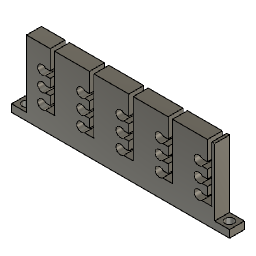
ESC Tray Holder v2 (Autodesk Fusion 360 design; units mm, degrees)
Autodesk Fusion 360 part; units mm, degrees
box "BoxPrimitive2" add length 25.4 width 76.2 height 2.54 placed x (0, 0, 1) y (1, 0, 0) z (0, 1, 0) at (0, 0, 0)
sketch "Sketch3" plane through (0, 2.54, 0) normal (0, 1, 0) x (-1, 0, 0)
  line L0 (0, 25.4) -> (-76.2, 25.4)
  line L1 (-76.2, 25.4) -> (-76.2, 0)
  line L2 (-76.2, 0) -> (0, 0)
  line L3 (0, 0) -> (0, 25.4)
  line L4 (-76.2, 12.7) -> (-72.39, 12.7)
  line L5 (-72.39, 12.7) -> (-72.39, 25.4)
  line L6 (-72.39, 25.4) -> (-69.215, 25.4)
  line L7 (-69.215, 25.4) -> (-69.215, 0)
  line L8 (-69.215, 0) -> (-72.39, 0)
  line L9 (-72.39, 12.7) -> (-72.39, 0)
  line L10 (-69.215, 12.7) -> (-59.055, 12.7)
  line L11 (-59.055, 12.7) -> (-59.055, 25.4)
  line L12 (-59.055, 25.4) -> (-55.88, 25.4)
  line L13 (-55.88, 25.4) -> (-55.88, 0)
  line L14 (-55.88, 0) -> (-59.055, 0)
  line L15 (-59.055, 12.7) -> (-59.055, 0)
  line L16 (-55.88, 12.7) -> (-45.72, 12.7)
  line L17 (-45.72, 12.7) -> (-45.72, 0)
  line L18 (-45.72, 0) -> (-42.545, 0)
  line L19 (-42.545, 0) -> (-42.545, 25.4)
  line L20 (-42.545, 25.4) -> (-45.72, 25.4)
  line L21 (-45.72, 12.7) -> (-45.72, 25.4)
  line L22 (-42.545, 12.7) -> (-32.385, 12.7)
  line L23 (-32.385, 12.7) -> (-32.385, 25.4)
  line L24 (-32.385, 25.4) -> (-29.21, 25.4)
  line L25 (-29.21, 25.4) -> (-29.21, 0)
  line L26 (-29.21, 0) -> (-32.385, 0)
  line L27 (-32.385, 0) -> (-32.385, 12.7)
  line L28 (-29.21, 12.7) -> (-19.05, 12.7)
  line L29 (-19.05, 12.7) -> (-19.05, 25.4)
  line L30 (-19.05, 25.4) -> (-15.875, 25.4)
  line L31 (-15.875, 25.4) -> (-15.875, 0)
  line L32 (-15.875, 0) -> (-19.05, 0)
  line L33 (-19.05, 0) -> (-19.05, 12.7)
  line L34 (-15.875, 12.7) -> (-12.065, 12.7)
  line L35 (-12.065, 12.7) -> (-12.065, 25.4)
  line L36 (-12.065, 12.7) -> (-12.065, 0)
  line L37 (-76.2, 12.7) -> (-76.2, 17.78)
  circle A0 centre (-70.8025, 17.78) radius 1.5875
  line L38 (-76.2, 12.7) -> (-76.2, 7.62)
  circle A1 centre (-70.8025, 7.62) radius 1.5875
  circle A2 centre (-70.8025, 12.7) radius 1.5875
  line L39 (-57.4675, 25.4) -> (-57.4675, 0)
  circle A3 centre (-57.4675, 12.7) radius 1.5875
  circle A4 centre (-57.4675, 17.78) radius 1.5875
  circle A5 centre (-57.4675, 7.62) radius 1.5875
  line L40 (-44.1325, 25.4) -> (-44.1325, 0)
  circle A6 centre (-44.1325, 12.7) radius 1.5875
  circle A7 centre (-44.1325, 17.78) radius 1.5875
  circle A8 centre (-44.1325, 7.62) radius 1.5875
  line L41 (-30.7975, 25.4) -> (-30.7975, 0)
  circle A9 centre (-30.7975, 12.7) radius 1.5875
  circle A10 centre (-30.7975, 7.62) radius 1.5875
  circle A11 centre (-30.7975, 17.78) radius 1.5875
  line L42 (-17.4625, 25.4) -> (-17.4625, 0)
  circle A12 centre (-17.4625, 12.7) radius 1.5875
  circle A13 centre (-17.4625, 17.78) radius 1.5875
  circle A14 centre (-17.4625, 7.62) radius 1.5875
  dimension "d17" = 3.81
  dimension "d18" = 3.175
  dimension "d19" = 3.175
  dimension "d20" = 10.16
  dimension "d21" = 3.175
  dimension "d22" = 3.175
  dimension "d23" = 10.16
  dimension "d24" = 3.175
  dimension "d25" = 3.175
  dimension "d26" = 10.16
  dimension "d27" = 3.175
  dimension "d28" = 3.175
  dimension "d29" = 10.16
  dimension "d30" = 3.175
  dimension "d31" = 3.175
  dimension "d32" = 3.81
  dimension "d37" = 5.08
  dimension "d38" = 3.175
  dimension "d39" = 5.08
  dimension "d40" = 3.175
  dimension "d41" = 3.175
  dimension "d42" = 3.175
  dimension "d43" = 3.175
  dimension "d44" = 3.175
  dimension "d45" = 3.175
  dimension "d46" = 3.175
  dimension "d47" = 3.175
  dimension "d48" = 3.175
  dimension "d49" = 3.175
  dimension "d50" = 3.175
  dimension "d51" = 3.175
  dimension "d52" = 3.175
  dimension "d53" = 3.175
  constraint midpoint L1 L4.start
  constraint perpendicular L1 L4
  constraint coincident L0 L5.end
  constraint perpendicular L0 L5
  constraint perpendicular L5 L6
  constraint coincident L2 L7.end
  constraint perpendicular L2 L7
  constraint perpendicular L7 L8
  constraint midpoint L7 L10.start
  constraint perpendicular L7 L10
  constraint coincident L0 L11.end
  constraint perpendicular L0 L11
  constraint coincident L0 L12.end
  constraint coincident L2 L13.end
  constraint perpendicular L2 L13
  constraint perpendicular L13 L14
  constraint midpoint L13 L16.start
  constraint perpendicular L13 L16
  constraint coincident L2 L17.end
  constraint perpendicular L14 L17
  constraint coincident L2 L18.end
  constraint coincident L0 L19.end
  constraint perpendicular L0 L19
  constraint perpendicular L19 L20
  constraint midpoint L19 L22.start
  constraint perpendicular L19 L22
  constraint coincident L0 L23.end
  constraint perpendicular L0 L23
  constraint coincident L0 L24.end
  constraint coincident L2 L25.end
  constraint perpendicular L2 L25
  constraint perpendicular L25 L26
  constraint midpoint L25 L28.start
  constraint perpendicular L25 L28
  constraint perpendicular L28 L29
  constraint perpendicular L29 L30
  constraint coincident L2 L31.end
  constraint perpendicular L2 L31
  constraint perpendicular L31 L32
  constraint midpoint L31 L34.start
  constraint perpendicular L31 L34
  constraint coincident L0 L35.end
  constraint perpendicular L0 L35
  constraint coincident L2 L36.end
  constraint perpendicular L2 L36
  constraint perpendicular L4 L37
  constraint perpendicular L4 L38
  constraint midpoint L12 L39.start
  constraint midpoint L14 L39.end
  constraint midpoint L39 A3.centre
  constraint coincident L39 A4.centre
  constraint coincident L39 A5.centre
  constraint midpoint L20 L40.start
  constraint midpoint L18 L40.end
  constraint midpoint L40 A6.centre
  constraint coincident L40 A7.centre
  constraint coincident L40 A8.centre
  constraint midpoint L24 L41.start
  constraint midpoint L26 L41.end
  constraint midpoint L41 A9.centre
  constraint coincident L41 A10.centre
  constraint coincident L41 A11.centre
  constraint midpoint L30 L42.start
  constraint midpoint L32 L42.end
  constraint midpoint L42 A12.centre
  constraint coincident L42 A13.centre
  constraint coincident L42 A14.centre
  measures "d17" distance of L4.start L4.end
  measures "d18" distance of L5.end L6.end
  measures "d19" distance of L7.end L8.end
  measures "d20" distance of L10.start L10.end
  measures "d21" distance of L11.end L12.end
  measures "d22" distance of L13.end L14.end
  measures "d23" distance of L16.start L16.end
  measures "d24" distance of L17.end L18.end
  measures "d25" distance of L19.end L20.end
  measures "d26" distance of L22.start L22.end
  measures "d27" distance of L23.end L24.end
  measures "d28" distance of L25.end L26.end
  measures "d29" distance of L28.start L28.end
  measures "d30" distance of L29.end L30.end
  measures "d31" distance of L31.end L32.end
  measures "d32" distance of L34.start L34.end
  measures "d37" distance of L4.start L37.end
  measures "d38" diameter of A0
  measures "d39" distance of L4.start L38.end
  measures "d40" diameter of A1
  measures "d41" diameter of A2
  measures "d42" diameter of A3
  measures "d43" diameter of A4
  measures "d44" diameter of A5
  measures "d45" diameter of A6
  measures "d46" diameter of A7
  measures "d47" diameter of A8
  measures "d48" diameter of A9
  measures "d49" diameter of A10
  measures "d50" diameter of A11
  measures "d51" diameter of A12
  measures "d52" diameter of A13
  measures "d53" diameter of A14
scale "Scale1" factors (0.841667, 1, 1) about (0, 2.54, 25.4) bodies 1
move_body "Move1" bodies 1 to x (1, 0, 0) y (0, 1, 0) z (0, 0, 1) at (12.065, 0, 0)
extrude "Extrude1" cut sketch "Sketch3" against normal blind 12.7 contours L42 A13 | L42 A12 | L42 A13 | L42 A14 | L42 A12 | L42 A14 | L41 A11 | L41 A9 | L41 A11 | L41 A10 | L41 A9 | L41 A10 | L40 A7 | L40 A6 | L40 A7 | L40 A8 | L40 A6 | L40 A8 | L39 A4 | L39 A3 | L39 A4 | L39 A5 | L39 A3 | L39 A5 | A0 | A2 | A1
sketch "Sketch4" plane through (76.2, 0, 0) normal (1, 0, 0) x (0, 1, 0)
  line L0 (2.54, 25.4) -> (0, 25.4)
  line L1 (0, 25.4) -> (0, 0)
  line L2 (0, 0) -> (2.54, 0)
  line L3 (2.54, 0) -> (2.54, 25.4)
  line L4 (2.54, 0) -> (2.54, 2.54)
  line L5 (0, 2.54) -> (2.54, 2.54)
  line L6 (0, 2.54) -> (0, 0)
  line L7 (2.54, 0) -> (0, 0)
  dimension "d56" = 2.54
  constraint coincident L2.end L3.start
  constraint coincident L3 L4.end
  constraint coincident L1 L5.start
  constraint perpendicular L4 L5
  constraint coincident L1.end L2.start
  measures "d56" distance of L2.end L4.end
extrude "Extrude2" add sketch "Sketch4" along normal blind 5.08 contours L1 L2 L3 L4 L5 L6 L7
sketch "Sketch5" plane through (12.065, 0, 0) normal (-1, 0, 0) x (0, -1, 0)
  line L0 (-2.54, 0) -> (0, 0)
  line L1 (0, 0) -> (0, 25.4)
  line L2 (0, 25.4) -> (-2.54, 25.4)
  line L3 (-2.54, 25.4) -> (-2.54, 0)
  line L4 (0, 0) -> (0, 2.54)
  line L5 (0, 2.54) -> (-2.54, 2.54)
  line L6 (-2.54, 0) -> (-2.54, 2.54)
  line L7 (-2.54, 0) -> (0, 0)
  dimension "d59" = 2.54
  constraint coincident L0.end L1.start
  constraint perpendicular L0 L4
  constraint coincident L3 L5.end
  constraint perpendicular L3 L5
  constraint coincident L0.start L3.end
  measures "d59" distance of L0.end L4.end
extrude "Extrude3" add sketch "Sketch5" along normal blind 5.08 contours L0 L1 L3 L4 L5 L6 L7
move_face "MoveFace1" by (0, 2.54, 0) 1 faces at (39.727, 2.54, 2.0123)
sketch "Sketch7" plane through (0, 0, 2.54) normal (0, 0, 1) x (-1, 0, 0)
  line L0 (-76.2, -5.08) -> (-76.2, 0)
  line L1 (-76.2, 0) -> (-81.28, 0)
  line L2 (-81.28, 0) -> (-81.28, -5.08)
  line L3 (-81.28, -5.08) -> (-76.2, -5.08)
  line L4 (-81.28, -5.08) -> (-81.28, -2.54)
  line L5 (-78.74, -2.54) -> (-78.74, -5.08)
  circle A0 centre (-78.74, -2.54) radius 1.5
  dimension "d63" = 3
  constraint coincident L2.end L3.start
  constraint midpoint L2 L4.end
  constraint midpoint L3 L5.end
  constraint perpendicular L3 L5
  constraint coincident L5.start A0.centre
  measures "d63" diameter of A0
sketch "Sketch8" plane through (0, 0, 2.54) normal (0, 0, 1) x (-1, 0, 0)
  line L0 (-12.065, 0) -> (-12.065, -5.08)
  line L1 (-12.065, -5.08) -> (-6.985, -5.08)
  line L2 (-6.985, -5.08) -> (-6.985, 0)
  line L3 (-6.985, 0) -> (-12.065, 0)
  line L4 (-6.985, -2.54) -> (-9.525, -2.54)
  circle A0 centre (-9.525, -2.54) radius 1.5
  dimension "d64" = 3
  constraint midpoint L2 L4.start
  constraint perpendicular L2 L4
  constraint coincident L4.end A0.centre
  measures "d64" diameter of A0
extrude "Extrude4" cut sketch "Sketch8" sketch "Sketch7" against normal blind 5 contours A0 of sketch 2 contours A0
sketch "Sketch9" plane through (0, 0, 0) normal (0, 1, 0) x (1, 0, 0)
  line L0 (18.6768, -18.816) -> (20.1542, -18.816)
  line L1 (20.1542, -18.816) -> (20.1542, -26.2967)
  line L2 (20.1542, -26.2967) -> (21.6542, -26.2967)
  line L3 (21.6542, -26.2967) -> (21.6542, -16.6091)
  line L4 (18.1034, -16.6091) -> (18.1034, -18.816)
  line L5 (18.1034, -18.816) -> (18.6768, -18.816)
  line L6 (18.1034, -11.5091) -> (18.1034, -13.716)
  line L7 (18.1034, -13.716) -> (18.6768, -13.716)
  line L8 (18.6768, -13.716) -> (20.1542, -13.716)
  line L9 (20.1542, -13.716) -> (20.1542, -16.6091)
  line L10 (20.1542, -16.6091) -> (18.1034, -16.6091)
  line L11 (18.1034, -8.616) -> (18.6768, -8.616)
  line L12 (18.6768, -8.616) -> (20.1542, -8.616)
  line L13 (21.6542, -6.4091) -> (18.1034, -6.4091)
  line L14 (18.1034, -6.4091) -> (18.1034, -8.616)
  line L15 (21.6542, -6.4091) -> (21.6542, -16.6091)
  line L16 (20.1542, -8.616) -> (20.1542, -11.5091)
  line L17 (20.1542, -11.5091) -> (18.1034, -11.5091)
  line L18 (35.0542, -26.2967) -> (35.0542, -16.6091)
  line L19 (33.5542, -26.2967) -> (35.0542, -26.2967)
  line L20 (33.5542, -18.816) -> (33.5542, -26.2967)
  line L21 (32.0768, -18.816) -> (33.5542, -18.816)
  line L22 (31.5034, -18.816) -> (32.0768, -18.816)
  line L23 (31.5034, -16.6091) -> (31.5034, -18.816)
  line L24 (33.5542, -16.6091) -> (31.5034, -16.6091)
  line L25 (33.5542, -13.716) -> (33.5542, -16.6091)
  line L26 (32.0768, -13.716) -> (33.5542, -13.716)
  line L27 (31.5034, -13.716) -> (32.0768, -13.716)
  line L28 (31.5034, -11.5091) -> (31.5034, -13.716)
  line L29 (33.5542, -11.5091) -> (31.5034, -11.5091)
  line L30 (33.5542, -8.616) -> (33.5542, -11.5091)
  line L31 (32.0768, -8.616) -> (33.5542, -8.616)
  line L32 (31.5034, -8.616) -> (32.0768, -8.616)
  line L33 (31.5034, -6.4091) -> (31.5034, -8.616)
  line L34 (35.0542, -6.4091) -> (31.5034, -6.4091)
  line L35 (35.0542, -6.4091) -> (35.0542, -16.6091)
  line L36 (48.4542, -26.2967) -> (48.4542, -16.6091)
  line L37 (46.9542, -26.2967) -> (48.4542, -26.2967)
  line L38 (46.9542, -18.816) -> (46.9542, -26.2967)
  line L39 (45.4768, -18.816) -> (46.9542, -18.816)
  line L40 (44.9034, -18.816) -> (45.4768, -18.816)
  line L41 (44.9034, -16.6091) -> (44.9034, -18.816)
  line L42 (46.9542, -16.6091) -> (44.9034, -16.6091)
  line L43 (46.9542, -13.716) -> (46.9542, -16.6091)
  line L44 (45.4768, -13.716) -> (46.9542, -13.716)
  line L45 (44.9034, -13.716) -> (45.4768, -13.716)
  line L46 (44.9034, -11.5091) -> (44.9034, -13.716)
  line L47 (46.9542, -11.5091) -> (44.9034, -11.5091)
  line L48 (46.9542, -8.616) -> (46.9542, -11.5091)
  line L49 (45.4768, -8.616) -> (46.9542, -8.616)
  line L50 (44.9034, -8.616) -> (45.4768, -8.616)
  line L51 (44.9034, -6.4091) -> (44.9034, -8.616)
  line L52 (48.4542, -6.4091) -> (44.9034, -6.4091)
  line L53 (48.4542, -6.4091) -> (48.4542, -16.6091)
  line L54 (61.8542, -6.4091) -> (61.8542, -16.6091)
  line L55 (61.8542, -6.4091) -> (58.3034, -6.4091)
  line L56 (58.3034, -6.4091) -> (58.3034, -8.616)
  line L57 (58.3034, -8.616) -> (58.8768, -8.616)
  line L58 (58.8768, -8.616) -> (60.3542, -8.616)
  line L59 (60.3542, -8.616) -> (60.3542, -11.5091)
  line L60 (60.3542, -11.5091) -> (58.3034, -11.5091)
  line L61 (58.3034, -11.5091) -> (58.3034, -13.716)
  line L62 (58.3034, -13.716) -> (58.8768, -13.716)
  line L63 (58.8768, -13.716) -> (60.3542, -13.716)
  line L64 (60.3542, -13.716) -> (60.3542, -16.6091)
  line L65 (60.3542, -16.6091) -> (58.3034, -16.6091)
  line L66 (58.3034, -16.6091) -> (58.3034, -18.816)
  line L67 (58.3034, -18.816) -> (58.8768, -18.816)
  line L68 (58.8768, -18.816) -> (60.3542, -18.816)
  line L69 (60.3542, -18.816) -> (60.3542, -26.2967)
  line L70 (60.3542, -26.2967) -> (61.8542, -26.2967)
  line L71 (61.8542, -26.2967) -> (61.8542, -16.6091)
  line L72 (75.2542, -26.2967) -> (75.2542, -16.6091)
  line L73 (73.7542, -26.2967) -> (75.2542, -26.2967)
  line L74 (73.7542, -18.816) -> (73.7542, -26.2967)
  line L75 (72.2768, -18.816) -> (73.7542, -18.816)
  line L76 (71.7034, -18.816) -> (72.2768, -18.816)
  line L77 (71.7034, -16.6091) -> (71.7034, -18.816)
  line L78 (73.7542, -16.6091) -> (71.7034, -16.6091)
  line L79 (73.7542, -13.716) -> (73.7542, -16.6091)
  line L80 (72.2768, -13.716) -> (73.7542, -13.716)
  line L81 (71.7034, -13.716) -> (72.2768, -13.716)
  line L82 (71.7034, -11.5091) -> (71.7034, -13.716)
  line L83 (73.7542, -11.5091) -> (71.7034, -11.5091)
  line L84 (73.7542, -8.616) -> (73.7542, -11.5091)
  line L85 (72.2768, -8.616) -> (73.7542, -8.616)
  line L86 (71.7034, -8.616) -> (72.2768, -8.616)
  line L87 (71.7034, -6.4091) -> (71.7034, -8.616)
  line L88 (75.2542, -6.4091) -> (71.7034, -6.4091)
  line L89 (75.2542, -6.4091) -> (75.2542, -16.6091)
  dimension "d67" = 1.5
  dimension "d74" = 1.5
  dimension "d75" = 1.5
  dimension "d76" = 1.5
  dimension "d77" = 1.5
  constraint horizontal L0
  constraint perpendicular L0 L1
  constraint perpendicular L1 L2
  constraint perpendicular L2 L3
  constraint perpendicular L0 L4
  constraint perpendicular L4 L5
  constraint horizontal L8
  constraint perpendicular L6 L8
  constraint perpendicular L6 L7
  constraint perpendicular L8 L9
  constraint perpendicular L4 L10
  constraint horizontal L12
  constraint perpendicular L12 L14
  constraint perpendicular L11 L14
  constraint perpendicular L13 L15
  constraint perpendicular L12 L16
  constraint perpendicular L6 L17
  constraint horizontal L21
  constraint perpendicular L20 L21
  constraint perpendicular L19 L20
  constraint perpendicular L18 L19
  constraint perpendicular L21 L23
  constraint perpendicular L22 L23
  constraint horizontal L26
  constraint perpendicular L26 L28
  constraint perpendicular L27 L28
  constraint perpendicular L25 L26
  constraint perpendicular L23 L24
  constraint horizontal L31
  constraint perpendicular L31 L33
  constraint perpendicular L32 L33
  constraint perpendicular L34 L35
  constraint perpendicular L30 L31
  constraint perpendicular L28 L29
  constraint horizontal L39
  constraint perpendicular L38 L39
  constraint perpendicular L37 L38
  constraint perpendicular L36 L37
  constraint perpendicular L39 L41
  constraint perpendicular L40 L41
  constraint horizontal L44
  constraint perpendicular L44 L46
  constraint perpendicular L45 L46
  constraint perpendicular L43 L44
  constraint perpendicular L41 L42
  constraint horizontal L49
  constraint perpendicular L49 L51
  constraint perpendicular L50 L51
  constraint perpendicular L52 L53
  constraint perpendicular L48 L49
  constraint perpendicular L46 L47
  constraint horizontal L68
  constraint perpendicular L68 L69
  constraint perpendicular L69 L70
  constraint perpendicular L70 L71
  constraint perpendicular L66 L68
  constraint perpendicular L66 L67
  constraint horizontal L63
  constraint perpendicular L61 L63
  constraint perpendicular L61 L62
  constraint perpendicular L63 L64
  constraint perpendicular L65 L66
  constraint horizontal L58
  constraint perpendicular L56 L58
  constraint perpendicular L56 L57
  constraint perpendicular L54 L55
  constraint perpendicular L58 L59
  constraint perpendicular L60 L61
  constraint horizontal L75
  constraint perpendicular L74 L75
  constraint perpendicular L73 L74
  constraint perpendicular L72 L73
  constraint perpendicular L75 L77
  constraint perpendicular L76 L77
  constraint horizontal L80
  constraint perpendicular L80 L82
  constraint perpendicular L81 L82
  constraint perpendicular L79 L80
  constraint perpendicular L77 L78
  constraint horizontal L85
  constraint perpendicular L85 L87
  constraint perpendicular L86 L87
  constraint perpendicular L88 L89
  constraint perpendicular L84 L85
  constraint perpendicular L82 L83
  measures "d67" distance of L1.end L2.end
  measures "d74" distance of L18.start L19.start
  measures "d75" distance of L36.start L37.start
  measures "d76" distance of L69.end L70.end
  measures "d77" distance of L72.start L73.start
extrude "Extrude5" cut sketch "Sketch9" along normal blind 11
